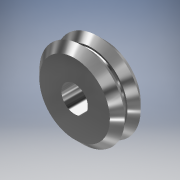
# Autodesk Inventor part: roller
Saved by Autodesk Inventor 2017 SP1 (Build 210196100, 196)
## iProperties
Created: 2018-01-18
Part Number: roller
Material: Steel, Alloy
Document SubType Name: Modeling
Designer: Ben
Density: 7.73 g/cm^3
Appearance: Chrome - Polished
Author: Ben
Autodesk Inventor part; units mm, degrees
ref_plane "YZ Plane" through (0, 0, 0) normal (1, 0, 0) x (0, 1, 0)
ref_plane "XZ Plane" through (0, 0, 0) normal (0, 1, 0) x (-1, 0, 0)
ref_plane "XY Plane" through (0, 0, 0) normal (0, 0, 1) x (1, 0, 0)
sketch "Sketch1" plane through (0, 0, 0) normal (1, 0, 0) x (0, 1, 0)
  line L0 (4.7625, 5.5372) -> (4.7625, -5.5372)
  line L1 (4.7625, 5.5372) -> (12.7, 5.5372)
  line L2 (12.7, 5.5372) -> (15.367, 2.8702)
  line L3 (15.367, -2.8702) -> (12.7, -5.5372)
  line L4 (12.7, -5.5372) -> (4.7625, -5.5372)
  line L5 (4.7625, 0) -> (0, 0) construction
  line L6 (4.7625, 0) -> (12.3952, 0) construction
  line L7 (15.367, 2.8702) -> (13.0048, 0.508)
  line L8 (13.0048, -0.508) -> (15.367, -2.8702)
  line L9 (13.0048, 0.508) -> (12.3952, 0.508)
  line L10 (12.3952, 0.508) -> (12.3952, -0.508)
  line L11 (12.3952, -0.508) -> (13.0048, -0.508)
  line L12 (0, -5.4393) -> (0, 5.4393) construction
  line L13 (12.7, 5.5372) -> (12.7, 0.508) construction
  dimension "d0" = 4.7625
  dimension "d1" = 12.7
  dimension "d3" = 1.016
  dimension "d4" = 11.0744
  dimension "d6" = 15.367
  dimension "d7" = 5.7404
  constraints: 28 end point, 5 horizontal, 5 perpendicular, 4 midpoint, 3 equal length, 3 vertical
  measures "d0" distance of L5.start L5.end
  measures "d1" horizontal distance of L5.end L1.end
  measures "d3" distance of L9.end L10.end
  measures "d4" distance of L0.start L0.end
  measures "d6" distance from line of L12 L3.start
  measures "d7" distance of L2.end L3.start
revolve "Revolution1" add sketch "Sketch1" angle 360 about axis through (0, 0, -5.4393) along (0, 0, 1)
body "Solid1"
